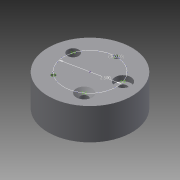
# Autodesk Inventor part: HolePracticeDE
Saved by Autodesk Inventor 2015 (Build 190159000, 159)
## iProperties
Created: 2017-12-12
Part Number: HolePracticeDE
Material: Generic
Document SubType Name: Modeling
Designer: Administrator
Density: 1 g/cm^3
Appearance: Default
Author: Administrator
Autodesk Inventor part; units mm, degrees
ref_plane "YZ Plane" through (0, 0, 0) normal (1, 0, 0) x (0, 1, 0)
ref_plane "XZ Plane" through (0, 0, 0) normal (0, 1, 0) x (-1, 0, 0)
ref_plane "XY Plane" through (0, 0, 0) normal (0, 0, 1) x (1, 0, 0)
sketch "Sketch1" plane through (0, 0, 0) normal (0, 1, 0) x (-1, 0, 0)
  circle A0 centre (0, 0) radius 50.8
  dimension "d0" = 101.6
  constraints: 1 centre point, 1 coincident
  measures "d0" diameter of A0
extrude "Extrusion1" add sketch "Sketch1" along normal blind 38.1
sketch "Sketch2" plane through (0, 38.1, 0) normal (0, 1, 0) x (1, 0, 0)
  circle A0 centre (0, 0) radius 31.75 construction
  point P0 (0, 31.75)
  point P1 (-30.196, 9.8113)
  point P2 (-18.6622, -25.6863)
  point P3 (18.6622, -25.6863)
  point P4 (30.196, 9.8113)
  dimension "d4" = 63.5
  dimension "d7" = 360
  constraints: 1 coincident, 1 vertical alignment, 8 other
hole "Hole1" at (0, 38.1, -31.75) direction (0, -1, 0) diameter 6.35 end through all
hole "Hole2" at (30.196, 38.1, -9.8113) direction (0, -1, 0) diameter 9.525 end through all counterbore diameter 19.05 counterbore depth 6.35
hole "Hole3" at (18.6622, 38.1, 25.6863) direction (0, -1, 0) diameter 9.525 end through all countersink diameter 19.05 countersink angle 82
hole "Hole4" at (-18.6622, 38.1, 25.6863) direction (0, -1, 0) diameter 4.9784 end through all thread size "1/4-20 UNC" class "1B" standard "ANSI Unified Screw Threads"
hole "Hole5" at (-30.196, 38.1, -9.8113) direction (0, -1, 0) diameter 13.4874 end through all clearance for "Flat Head Machine Screw (82)" size "1/2" standard "Ansi Unified Screw Threads"
body "Solid1"
